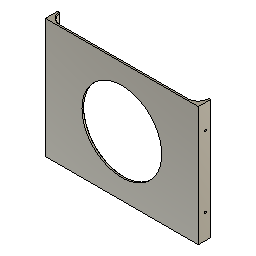
support_étagères_230 (Autodesk Fusion 360 design; units mm, degrees)
Autodesk Fusion 360 part; units mm, degrees
sketch "Esquisse1" plane through (0, 0, 0) normal (0, 1, 0) x (1, 0, 0)
  line L0 (130, 40) -> (-100, 40)
  line L1 (-100, 40) -> (-100, -140)
  line L2 (-100, -140) -> (130, -140)
  line L3 (130, -140) -> (130, 40)
  line L4 (130, 40) -> (-100, -140) construction
  line L5 (-100, 40) -> (130, -140) construction
  line L6 (-100, -140) -> (-85, -140)
  line L7 (-85, -140) -> (-85, 40)
  line L8 (-85, 40) -> (-100, 40)
  line L9 (-100, 40) -> (-100, -140)
  line L10 (130, -140) -> (115, -140)
  line L11 (115, -140) -> (115, 40)
  line L12 (115, 40) -> (130, 40)
  line L13 (130, 40) -> (130, -140)
  line L14 (-100, -140) -> (99.8736, -140)
  circle A0 centre (15, -50) radius 60
  line L15 (-100, 40) -> (100, 40)
  line L16 (100, 40) -> (100, 25)
  point P0 (15, -50)
  dimension "d1" = 230
  dimension "d2" = 180
  dimension "d3" = 15
  dimension "d4" = 15
  dimension "d12" = 120
  dimension "d13" = 115
  constraint horizontal L0
  constraint perpendicular L0 L1
  constraint parallel L0 L2
  constraint parallel L1 L3
  constraint coincident L4 P0
  constraint coincident L5 P0
  constraint horizontal L6
  constraint vertical L7
  constraint horizontal L8
  constraint vertical L9
  constraint coincident L0 L7.end
  constraint horizontal L10
  constraint vertical L11
  constraint horizontal L12
  constraint vertical L13
  constraint horizontal L14
  constraint horizontal L15
  measures "d1" distance of L1.end L2.end
  measures "d2" distance of L0.end L1.end
  measures "d3" distance of L1 L7
  measures "d4" distance of L2.end L10.end
  measures "d12" diameter of A0
  measures "d13" distance of L3 P0
extrude "Extrusion1" add sketch "Esquisse1" along normal blind 3.5
extrude "Extrusion4" add sketch "Esquisse1" along normal blind 18.5 contours L0 L2 L3 L10 L11 L12 L13 | L0 L1 L2 L6 L7 L8 L9 L14 L15
sketch "Esquisse5" plane through (115, 0, 0) normal (-1, 0, 0) x (0, -1, 0)
  line L0 (-3.5, -40) -> (-3.5, 140)
  line L1 (-3.5, 140) -> (-18.5, 140)
  line L2 (-18.5, 140) -> (-18.5, -40)
  line L3 (-18.5, -40) -> (-3.5, -40)
  circle A0 centre (-10.75, -3) radius 1.5
  circle A1 centre (-10.75, -3) radius 3.75
  circle A2 centre (-10.75, 103) radius 1.5
  circle A3 centre (-10.75, 103) radius 3.75
  dimension "d74" = 2.25
  dimension "d75" = 3
  dimension "d77" = 7.25
  dimension "d78" = 37
  dimension "d79" = 3
  dimension "d80" = 2.25
  dimension "d81" = 7.25
  dimension "d82" = 37
  measures "d75" diameter of A0
  measures "d77" distance of L0 A0.centre
  measures "d78" distance of L3 A0.centre
  measures "d79" diameter of A2
  measures "d81" distance of L0 A2.centre
  measures "d82" distance of L1 A2.centre
extrude "Extrusion9" cut sketch "Esquisse5" against normal blind 18.5 contours A0 | A2
extrude "Extrusion10" cut sketch "Esquisse5" against normal blind 11.5 contours A1 | A3
sketch "Esquisse3" plane through (0, 0, 140) normal (0, 0, 1) x (-1, 0, 0)
  line L0 (-115, -3.5) -> (85, -3.5)
  line L1 (85, -3.5) -> (85, -18.5)
  line L2 (85, -18.5) -> (100, -18.5)
  line L3 (100, -18.5) -> (100, 0)
  line L4 (100, 0) -> (-130, 0)
  line L5 (-130, 0) -> (-130, -18.5)
  line L6 (-130, -18.5) -> (-115, -18.5)
  line L7 (-115, -18.5) -> (-115, -3.5)
  circle A0 centre (-111.5, -18.5) radius 15
  line L8 (-99.5, -19) -> (-85, -19)
  line L9 (-85, -19) -> (-85, -4)
  line L10 (-99.5, 0) -> (-99.5, -19)
  circle A1 centre (81.5, -18.5) radius 15
  dimension "d28" = 30
  dimension "d29" = 15
  dimension "d30" = 18.5
  dimension "d33" = 30
  dimension "d34" = 15
  dimension "d35" = 18.5
  measures "d28" diameter of A0
  measures "d29" distance of L0 A0.centre
  measures "d30" distance of L5 A0.centre
  measures "d33" diameter of A1
  measures "d34" distance of L0 A1.centre
  measures "d35" distance of L2.end A1.centre
extrude "Extrusion5" cut sketch "Esquisse3" against normal blind 180 contours L6 L7 A0 L8 L10 | L6 L7 A0 | L1 L2 A1 picked at (92.6117, -17.7609)
sketch "Esquisse4" plane through (130, 0, 0) normal (1, 0, 0) x (0, 1, 0)
  line L0 (0, 140) -> (0, -40)
  line L1 (0, -40) -> (18.5, -40)
  line L2 (18.5, -40) -> (18.5, 140)
  line L3 (18.5, 140) -> (0, 140)
  line L4 (18.5, 130.75) -> (0, 130.75)
  line L5 (0, 130.75) -> (0, 112.25)
  line L6 (0, 112.25) -> (18.5, 112.25)
  line L7 (18.5, 112.25) -> (18.5, 130.75)
  line L8 (18.5, -30.75) -> (0, -30.75)
  line L9 (0, -30.75) -> (0, -12.25)
  line L10 (0, -12.25) -> (18.5, -12.25)
  line L11 (18.5, -12.25) -> (18.5, -30.75)
  circle A0 centre (10.375, -21.5) radius 3.0833
  line L12 (10.8993, -18.4616) -> (0, -12.25)
  line L13 (10.8362, -24.5486) -> (0, -30.75)
  circle A1 centre (10.375, 121.5) radius 3.0833
  line L14 (0, 130.75) -> (11.8653, 124.1993)
  line L15 (11.8653, 118.8007) -> (0, 112.25)
  line L16 (0, -40) -> (0, 140)
  circle A2 centre (10.75, 103) radius 1.5
  circle A3 centre (10.75, -3) radius 1.5
  dimension "d38" = 18.5
  dimension "d39" = 9.25
  dimension "d40" = 18.5
  dimension "d41" = 18.5
  dimension "d42" = 9.25
  dimension "d43" = 6.1667
  dimension "d46" = 10.375
  dimension "d49" = 6.1667
  dimension "d50" = 9.25
  dimension "d54" = 10.375
  dimension "d55" = 9.25
  dimension "d91" = 18.5
  constraint horizontal L4
  constraint vertical L5
  constraint horizontal L6
  constraint vertical L7
  constraint coincident L2 L4.start
  constraint horizontal L8
  constraint vertical L9
  constraint horizontal L10
  constraint vertical L11
  constraint coincident L2 L8.start
  constraint coincident A0 L12.start
  constraint coincident A0 L13.start
  constraint coincident A1 L14.end
  constraint tangent A1 L14
  constraint coincident A1 L15.start
  constraint tangent A1 L15
  measures "d38" distance of L4.start L6.end
  measures "d39" distance of L3 L4.start
  measures "d40" distance of L8.start L10.end
  measures "d41" distance of L9 L11
  measures "d42" distance of L1 L8.start
  measures "d43" diameter of A0
  measures "d46" distance of L9 A0.centre
  measures "d49" diameter of A1
  measures "d50" distance of L4 A1.centre
  measures "d54" distance of A1.centre L16
  measures "d55" distance of L8 A0.centre
  measures "d91" distance of L5 L7
extrude "Extrusion6" add sketch "Esquisse4" against normal blind 230 contours L0 L9 A0 L12 L13 L16 | A0
extrude "Extrusion7" add sketch "Esquisse4" against normal blind 230 contours L0 L5 A1 L14 L15 L16 | A1
fillet "Congé1" radius 1 8 edges at (126.5, 18.5, 50) (-96.5, 18.5, 50) (15, 3.5, -40) (-93.2792, 9.2129, -40) (123.2792, 9.2129, 140) (123.2792, 9.2129, -40) (-93.2792, 9.2129, 140) (15, 3.5, 140)
fillet "Congé2" radius 1 1 edges at (-40.9396, 3.5, 28.3031)
equation "d1 = hauteur"
equation "d2 = profondeur"
equation "d3 = largeur_base"
equation "d4 = largeur_base"
equation "hauteur = 230 mm"
equation "profondeur = 180 mm"
equation "largeur_base = 15 mm"
equation "hauteur_nervure = 15 mm"
equation "diametre_trou = profondeur * 2 / 3"
equation "epaisseur_mini = 3.5 mm"
equation "d12 = diametre_trou"
equation "d13 = hauteur / 2"
equation "d15 = epaisseur_mini"
equation "epaisseur_nervure_base = epaisseur_mini + 15 mm"
equation "arc_congés = 1 mm"
equation "d25 = epaisseur_nervure_base"
equation "d28 = largeur_base * 2"
equation "d29 = largeur_base"
equation "d30 = largeur_base + epaisseur_mini"
equation "d33 = largeur_base * 2"
equation "d34 = largeur_base"
equation "d35 = largeur_base + epaisseur_mini"
equation "d36 = -profondeur"
equation "d38 = epaisseur_nervure_base"
equation "d39 = epaisseur_nervure_base / 2"
equation "d40 = epaisseur_nervure_base"
equation "d41 = epaisseur_nervure_base"
equation "d42 = epaisseur_nervure_base / 2"
equation "d43 = epaisseur_nervure_base / 3"
equation "d46 = epaisseur_nervure_base * 3 / 4 - epaisseur_mini"
equation "d47 = -hauteur"
equation "d49 = epaisseur_nervure_base / 3"
equation "d50 = epaisseur_nervure_base / 2"
equation "d52 = -hauteur"
equation "d54 = epaisseur_nervure_base * 3 / 4 - epaisseur_mini"
equation "d55 = epaisseur_nervure_base / 2"
equation "dia_vis = 3 mm"
equation "dia_lamage_vis = dia_vis + 1.5 * dia_vis"
equation "d74 = ( dia_lamage_vis - dia_vis ) / 2"
equation "d75 = dia_vis"
equation "d77 = epaisseur_mini + dia_lamage_vis / 2"
equation "d78 = epaisseur_nervure_base * 2"
equation "d79 = dia_vis"
equation "d80 = ( dia_lamage_vis - dia_vis ) / 2"
equation "d81 = d77"
equation "d82 = d78"
equation "d83 = -epaisseur_nervure_base"
equation "d85 = -epaisseur_nervure_base + epaisseur_mini * 2"
equation "d88 = arc_congés"
equation "d90 = arc_congés"
equation "d91 = epaisseur_nervure_base"
